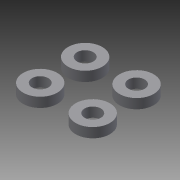
# Autodesk Inventor part: Washers
Saved by Autodesk Inventor 2014 SP1 (Build 180222100, 222)
## iProperties
Created: 2015-03-02
Part Number: Washers
Material: Generic
Document SubType Name: Modeling
Designer: Erin
Density: 1 g/cm^3
Appearance: Default
Author: Erin
Autodesk Inventor part; units mm, degrees
ref_plane "YZ Plane" through (0, 0, 0) normal (1, 0, 0) x (0, 1, 0)
ref_plane "XZ Plane" through (0, 0, 0) normal (0, 1, 0) x (-1, 0, 0)
ref_plane "XY Plane" through (0, 0, 0) normal (0, 0, 1) x (1, 0, 0)
sketch "Sketch1" plane through (0, 0, 0) normal (0, 0, 1) x (1, 0, 0)
  circle A0 centre (-7.0307, 6.2672) radius 2.25
  circle A1 centre (-7.0307, 6.2672) radius 4.75
  circle A2 centre (6.649, 6.8398) radius 2.25
  circle A3 centre (6.649, 6.8398) radius 4.75
  circle A4 centre (-7.0307, -6.2036) radius 2.25
  circle A5 centre (-7.0307, -6.2036) radius 4.75
  circle A6 centre (7.5397, -6.2036) radius 2.25
  circle A7 centre (7.5397, -6.2036) radius 4.75
  point P0 (0, 0)
  dimension "d0" = 4.5
  dimension "d1" = 2.5
  dimension "d2" = 4.5
  dimension "d3" = 2.5
  dimension "d4" = 4.5
  dimension "d5" = 2.5
  dimension "d6" = 4.5
  dimension "d7" = 2.5
  constraints: 8 centre point, 4 coincident
  measures "d0" diameter of A0
  measures "d1" radial gap between concentric circles of A0 A1
  measures "d2" diameter of A2
  measures "d3" radial gap between concentric circles of A2 A3
  measures "d4" diameter of A4
  measures "d5" radial gap between concentric circles of A4 A5
  measures "d6" diameter of A6
  measures "d7" radial gap between concentric circles of A6 A7
extrude "Extrusion1" add sketch "Sketch1" along normal blind 2.7
body "Solid1"
